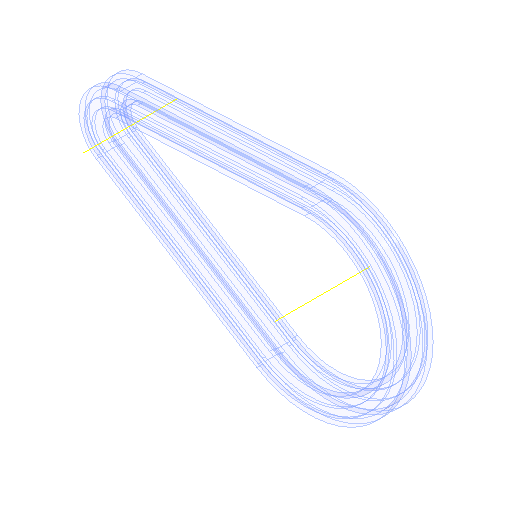
# Autodesk Inventor part: Roller Chain
Saved by Autodesk Inventor 2024 (Build 280153000, 153)
## iProperties
Created: 2024-02-29
Part Number: Roller Chain
Material: Generic
Document SubType Name: Modeling
Designer: seene
Density: 1 g/cm^3
Appearance: Clear - Blue
CustomPartVersion: 1
Author: seene
Autodesk Inventor part; units mm, degrees
ref_plane "Work Plane2" through (-96.619782, 62.868773, 0) normal (-1, 0, 0) x (0, 0, 1)
ref_plane "Work Plane3" through (-0.2675, 37.944761, 0) normal (-0.9927601, 0.120114, 0) x (0, 0, 1)
sketch "Path" plane through (0, 0, 0) normal (0, 0, 1) x (1, 0, 0)
  arc A0 (-97.280817, 75.551558) -> (-103.347849, 52.097371) centre (-96.619782, 62.868773) ccw
  arc A1 (-22.838506, 1.809367) -> (-2.48511, 80.492373) centre (-0.2675, 37.944761) ccw
  line L0 (-22.838506, 1.809367) -> (-103.347849, 52.097371)
  line L1 (-97.280817, 75.551558) -> (-2.48511, 80.492373)
  dimension "d31" = 11.9888
  constraints: 4 end point, 4 point on circle, 2 centre point
ref_plane "Section Plane" through (-103.347849, 52.097371, 0) normal (0.8481419, -0.5297691, 0) x (0, 0, 1)
sketch "Section Sketch" plane through (-103.347849, 52.097371, 0) normal (0.8481419, -0.5297691, 0) x (0, 0, 1)
  line L0 (-8.509, -1.9812) -> (8.509, -1.9812)
  line L1 (8.509, -1.9812) -> (8.509, 1.9812)
  line L2 (8.509, 1.9812) -> (-8.509, 1.9812)
  line L3 (-8.509, 1.9812) -> (-8.509, -1.9812)
  line L4 (-3.9624, -3.9624) -> (3.9624, -3.9624)
  line L5 (3.9624, -3.9624) -> (3.9624, 3.9624)
  line L6 (3.9624, 3.9624) -> (-3.9624, 3.9624)
  line L7 (-3.9624, 3.9624) -> (-3.9624, -3.9624)
  line L8 (-3.9624, 0) -> (3.9624, 0) construction
  line L9 (-7.0104, -5.9944) -> (-3.9624, -5.9944)
  line L10 (-3.9624, -5.9944) -> (-3.9624, 5.9944)
  line L11 (-3.9624, 5.9944) -> (-7.0104, 5.9944)
  line L12 (-7.0104, 5.9944) -> (-7.0104, -5.9944)
  line L13 (3.9624, -5.9944) -> (7.0104, -5.9944)
  line L14 (7.0104, -5.9944) -> (7.0104, 5.9944)
  line L15 (7.0104, 5.9944) -> (3.9624, 5.9944)
  line L16 (3.9624, 5.9944) -> (3.9624, -5.9944)
  line L17 (-8.509, 0) -> (8.509, 0) construction
  point P0 (0, 0)
  point P1 (0, 0)
  dimension "d21" = 3.9624
  dimension "d22" = 7.9248
  dimension "d23" = 7.9248
  dimension "d24" = 3.048
  dimension "d31" = 11.9888
  dimension "d32" = 17.018
  constraints: 36 end point, 8 midpoint, 8 parallel, 4 horizontal, 4 perpendicular, 3 collinear, 1 coincident, 1 other
  measures "d21" distance between parallel lines of L2 L0
  measures "d22" distance between parallel lines of L6 L4
  measures "d23" distance between parallel lines of L5 L7
  measures "d24" distance between parallel lines of L12 L10
  measures "d31" distance between parallel lines of L11 L9
  measures "d32" distance between parallel lines of L1 L3
sweep "Solid" add profiles "Section Sketch" path "Path"
pattern_of_one "Strand Pattern"
equation "\"d21\" = da_d2"
equation "\"d22\" = da_d1"
equation "\"d23\" = da_b1"
equation "\"d24\" = da_t1 + da_t2"
equation "\"d30\" = da_pt"
equation "\"da_p\" = 12.7"
equation "\"da_b1\" = 7.9248"
equation "\"da_h2\" = 11.9888"
equation "\"da_h3\" = 10.3886"
equation "\"da_d1\" = 7.9248"
equation "\"da_d2\" = 3.9624"
equation "\"da_pt\" = 14.3764"
equation "\"da_b\" = 17.018"
equation "\"da_t1\" = 1.524"
equation "\"da_t2\" = 1.524"
body "Solid1"
